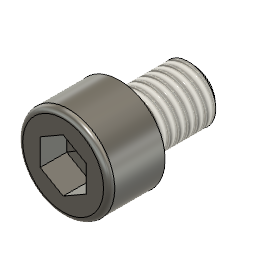
SDS Idler Tube Plug (Autodesk Fusion 360 archive; units mm, degrees)
design "Hexagon Socket Head Cap Screw ANSI B18.3 - 10-32 UNF x 1/4 Steel Grade 2 Plain"
description: Hexagon Socket Head Cap Screw ANSI B18.3 - 10-32 UNF x 1/4
part number: HSHCS ANSI B18.3 - 10-32 UNF x 1/4 Steel Grade 2 Plain
Autodesk Fusion 360 part; units mm, degrees
sketch "Sketch1" plane through (0, 0, 0) normal (0, 1, 0) x (1, 0, 0)
  line L0 (-2.413, 0) -> (-2.413, 6.35)
  line L1 (-2.413, 6.35) -> (0, 6.35)
  line L2 (0, 6.35) -> (0, -4.826)
  line L3 (-2.413, 0) -> (-3.9624, 0)
  line L4 (-3.9624, 0) -> (-3.9624, -4.826)
  line L5 (-3.9624, -4.826) -> (0, -4.826)
  dimension "d107" = 4.826
  dimension "d108" = 6.35
  dimension "d114" = 7.9248
  dimension "d115" = 4.826
  constraint perpendicular L0 L1
  constraint collinear origin L1.end L2.end
  constraint perpendicular L0 L3
  constraint coincident origin L3
  constraint vertical L2
  constraint coincident L2 L5.end
  constraint perpendicular L2 L5
  measures "d107" distance of L3.end L5
  measures "d108" distance of origin L1
revolve "Revolve1" add sketch "Sketch1" angle 360 about axis through (0, 0, -6.35) along (0, 0, 1)
ref_plane "WorkPlane1" through (0, 0, 4.826) normal (0, 0, 1) x (1, 0, 0)
sketch "Sketch6" plane through (0, 0, 4.826) normal (0, 0, 1) x (1, 0, 0)
  line L0 (-1.9812, 1.1438) -> (-1.9812, -1.1438)
  line L1 (-1.9812, -1.1438) -> (0, -2.2877)
  line L2 (0, -2.2877) -> (1.9812, -1.1438)
  line L3 (1.9812, -1.1438) -> (1.9812, 1.1438)
  line L4 (1.9812, 1.1438) -> (0, 2.2877)
  line L5 (0, 2.2877) -> (-1.9812, 1.1438)
  dimension "d116" = 3.9624
  constraint vertical L3
  measures "d116" distance of L0 L3
extrude "Extrude1" cut sketch "Sketch6" against normal blind 2.286
extrude "Extrude2" cut 1 faces at (-0.6604, 0.3813, 2.54) along direction (0, 0, -1) blind 2.286 draft -85
thread "Thread3" "ANSI Unified Screw Threads 0.19(#10) 10-32 UNF 10-32 UNF 2A" major diameter 4.7269 minor diameter 3.8583 pitch 0.7937 angle 60 resizes the face on face at (-2.401, 0.2403, -4.2333) from (0, 0, -1.2365) to (0, 0, -6.35)
fillet "Fillet4" radius 0.4826 1 edges at (-3.6943, 1.4329, 4.826)
sketch "Sketch7" plane through (0, 0, 0) normal (0, 1, 0) x (1, 0, 0)
  line L0 (-2.4613, 6.35) -> (-2.4613, 5.8776)
  line L1 (-2.4613, 5.8776) -> (-1.9406, 6.35)
  line L2 (0, 6.35) -> (0, -4.826)
  line L3 (-2.4613, 6.35) -> (0, 6.35)
  dimension "d103" = 2.4613
  dimension "d110" = 1.9406
  dimension "d111" = 0.4724
  constraint coincident L2.start L3.end
  constraint perpendicular L2 L3
  constraint coincident L1.end L3
  constraint perpendicular L0 L3
  measures "d103" distance of origin L0
  measures "d110" distance of L1.end L2
  measures "d111" distance of L0.end L3
revolve "Revolve3" cut sketch "Sketch7" angle 360 about axis through (0, 0, 1.75) along (0, 0, 1)
equation "d31 = -adsk_phildepth"
equation "d71 = adsk_headh"
equation "d76 = -adsk_phildepth"
equation "adsk_nomlen = 0.25 in"
equation "adsk_headh = 0.19 in"
equation "adsk_headdia = 0.312 in"
equation "adsk_nomdia = 0.19 in"
equation "adsk_philwidth = 0.156 in"
equation "adsk_phildepth = 0.09 in"
equation "adsk_thrlen = 0.20132 in"
equation "d93 = adsk_nomdia * 0.1"
equation "adsk_startlen = 0.0186 in"
equation "adsk_endpointdia = 0.1528 in"
equation "d103 = adsk_nomdia * 0.51"
equation "d107 = adsk_headh"
equation "d108 = adsk_nomlen"
equation "d110 = adsk_endpointdia / 2"
equation "d111 = adsk_startlen"
equation "d113 = min(adsk_thrlen; adsk_nomlen - 0.001 mm)"
equation "d114 = adsk_headdia"
equation "d115 = adsk_nomdia"
equation "d116 = adsk_philwidth"

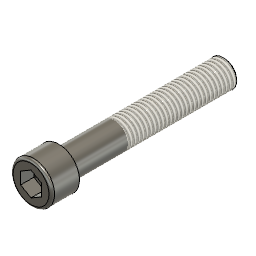
design "Hexagon Socket Head Cap Screw ANSI B18.3 - 1/4-28 UNF x 1 1/2 Steel Grade 2 Plain"
description: Hexagon Socket Head Cap Screw ANSI B18.3 - 1/4-28 UNF x 1 1/2
part number: HSHCS ANSI B18.3 - 1/4-28 UNF x 1 1/2 Steel Grade 2 Plain
Autodesk Fusion 360 part; units mm, degrees
sketch "Sketch1" plane through (0, 0, 0) normal (0, 1, 0) x (1, 0, 0)
  line L0 (-3.175, 0) -> (-3.175, 38.1)
  line L1 (-3.175, 38.1) -> (0, 38.1)
  line L2 (0, 38.1) -> (0, -6.35)
  line L3 (-3.175, 0) -> (-4.7625, 0)
  line L4 (-4.7625, 0) -> (-4.7625, -6.35)
  line L5 (-4.7625, -6.35) -> (0, -6.35)
  dimension "d107" = 6.35
  dimension "d108" = 38.1
  dimension "d114" = 9.525
  dimension "d115" = 6.35
  constraint perpendicular L0 L1
  constraint collinear origin L1.end L2.end
  constraint perpendicular L0 L3
  constraint coincident origin L3
  constraint vertical L2
  constraint coincident L2 L5.end
  constraint perpendicular L2 L5
  measures "d107" distance of L3.end L5
  measures "d108" distance of origin L1
revolve "Revolve1" add sketch "Sketch1" angle 360 about axis through (0, 0, -38.1) along (0, 0, 1)
ref_plane "WorkPlane1" through (0, 0, 6.35) normal (0, 0, 1) x (1, 0, 0)
sketch "Sketch6" plane through (0, 0, 6.35) normal (0, 0, 1) x (1, 0, 0)
  line L0 (-2.3876, 1.3785) -> (-2.3876, -1.3785)
  line L1 (-2.3876, -1.3785) -> (0, -2.757)
  line L2 (0, -2.757) -> (2.3876, -1.3785)
  line L3 (2.3876, -1.3785) -> (2.3876, 1.3785)
  line L4 (2.3876, 1.3785) -> (0, 2.757)
  line L5 (0, 2.757) -> (-2.3876, 1.3785)
  dimension "d116" = 4.7752
  constraint vertical L3
  measures "d116" distance of L0 L3
extrude "Extrude1" cut sketch "Sketch6" against normal blind 3.048
extrude "Extrude2" cut 1 faces at (0, 0.919, 3.302) along direction (0, 0, -1) blind 3.048 draft -85
thread "Thread3" "ANSI Unified Screw Threads 0.25 1/4-28 UNF 1/4-28 UNF 2A" major diameter 6.2433 minor diameter 5.2426 pitch 0.9071 angle 60 resizes the face on face at (-3.1592, 0.3161, -25.4) from (0, 0, -12.7) to (0, 0, -38.1)
fillet "Fillet4" radius 0.635 1 edges at (-4.4402, 1.7222, 6.35)
sketch "Sketch7" plane through (0, 0, 0) normal (0, 1, 0) x (1, 0, 0)
  line L0 (-3.2385, 38.1) -> (-3.2385, 37.559)
  line L1 (-3.2385, 37.559) -> (-2.634, 38.1)
  line L2 (0, 38.1) -> (0, -6.35)
  line L3 (-3.2385, 38.1) -> (0, 38.1)
  dimension "d103" = 3.2385
  dimension "d110" = 2.634
  dimension "d111" = 0.541
  constraint coincident L2.start L3.end
  constraint perpendicular L2 L3
  constraint coincident L1.end L3
  constraint perpendicular L0 L3
  measures "d103" distance of origin L0
  measures "d110" distance of L1.end L2
  measures "d111" distance of L0.end L3
revolve "Revolve3" cut sketch "Sketch7" angle 360 about axis through (0, 0, 1.75) along (0, 0, 1)
equation "d31 = -adsk_phildepth"
equation "d71 = adsk_headh"
equation "d76 = -adsk_phildepth"
equation "adsk_nomlen = 1.50 in"
equation "adsk_headh = 0.25 in"
equation "adsk_headdia = 0.375 in"
equation "adsk_nomdia = 0.25 in"
equation "adsk_philwidth = 0.188 in"
equation "adsk_phildepth = 0.12 in"
equation "adsk_thrlen = 1.00 in"
equation "d93 = adsk_nomdia * 0.1"
equation "adsk_startlen = 0.0213 in"
equation "adsk_endpointdia = 0.2074 in"
equation "d103 = adsk_nomdia * 0.51"
equation "d107 = adsk_headh"
equation "d108 = adsk_nomlen"
equation "d110 = adsk_endpointdia / 2"
equation "d111 = adsk_startlen"
equation "d113 = min(adsk_thrlen; adsk_nomlen - 0.001 mm)"
equation "d114 = adsk_headdia"
equation "d115 = adsk_nomdia"
equation "d116 = adsk_philwidth"
